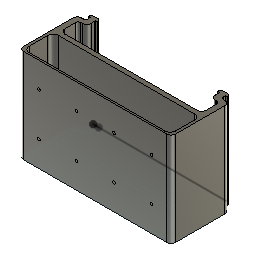
Robot Arm Holder (Autodesk Fusion 360 design; units mm, degrees)
Autodesk Fusion 360 part; units mm, degrees
sketch "Sketch1" plane through (0, 0, 0) normal (0, 0, 1) x (1, 0, 0)
  line L0 (69.451, 50) -> (67.151, 50)
  line L1 (-69.451, 50) -> (-67.151, 50)
  line L2 (-67.151, 50) -> (-67.151, 51)
  line L3 (-67.151, 51) -> (-69.4845, 53.3335)
  line L4 (-67.151, 51) -> (-63.851, 51) construction
  line L5 (-69.4845, 53.3335) -> (-75.6165, 53.3335)
  line L6 (-75.6165, 53.3335) -> (-77.9499, 51)
  line L7 (-75.6165, 53.3335) -> (-72.3165, 53.3335) construction
  line L8 (-77.9499, 51) -> (-77.9499, 50)
  line L9 (-77.9499, 50) -> (-75.6499, 50)
  line L10 (-75.6499, 50) -> (-75.6499, 47.5)
  line L11 (-85, -15) -> (-85, 40)
  arc A0 (-78.1499, 45) -> (-75.6499, 47.5) centre (-78.1499, 47.5) ccw
  arc A1 (-80, 45) -> (-85, 40) centre (-80, 40) ccw
  line L12 (-80, 45) -> (-78.1499, 45)
  line L13 (-80, -20) -> (80, -20)
  line L14 (85, -15) -> (85, 40)
  arc A2 (-85, -15) -> (-80, -20) centre (-80, -15) ccw
  arc A3 (80, -20) -> (85, -15) centre (80, -15) ccw
  arc A4 (85, 40) -> (80, 45) centre (80, 40) ccw
  arc A5 (-79, -12) -> (-76, -15) centre (-76, -12) ccw
  arc A6 (76, -15) -> (79, -12) centre (76, -12) ccw
  line L15 (76, -15) -> (-76, -15)
  arc A7 (-76, 40) -> (-79, 37) centre (-76, 37) ccw
  line L16 (-79, 37) -> (-79, -12)
  line L17 (79, -12) -> (79, 37)
  arc A8 (79, 37) -> (76, 40) centre (76, 37) ccw
  line L18 (80, 45) -> (78.15, 45)
  line L19 (75.65, 47.5) -> (75.65, 50)
  line L20 (75.65, 50) -> (77.95, 50)
  line L21 (77.95, 50) -> (77.95, 51)
  line L22 (77.95, 51) -> (75.6165, 53.3335)
  arc A9 (75.65, 47.5) -> (78.15, 45) centre (78.15, 47.5) ccw
  line L23 (75.6165, 53.3335) -> (69.4845, 53.3335)
  line L24 (69.4845, 53.3335) -> (67.1511, 51)
  line L25 (69.4845, 53.3335) -> (72.7845, 53.3335) construction
  line L26 (67.1511, 51) -> (67.151, 50)
  line L27 (69.451, 50) -> (69.451, 47.5)
  arc A10 (66.951, 45) -> (69.451, 47.5) centre (66.951, 47.5) ccw
  line L28 (-69.451, 50) -> (-69.451, 47.5)
  arc A11 (-69.451, 47.5) -> (-66.951, 45) centre (-66.951, 47.5) ccw
  line L29 (-66.951, 45) -> (66.951, 45)
  line L30 (-76, 40) -> (76, 40)
  dimension "d7" = 2.3
  dimension "d8" = 2.3
  dimension "d10" = 1
  dimension "d11" = 135
  dimension "d12" = 3.3
  dimension "d13" = 6.132
  dimension "d14" = 135
  dimension "d15" = 3.3
  dimension "d16" = 1
  dimension "d17" = 2.3
  dimension "d19" = 1.85
  dimension "d22" = 2.3
  dimension "d23" = 135
  dimension "d24" = 3.3
  dimension "d25" = 6.132
  dimension "d26" = 135
  dimension "d27" = 3.3
  constraint perpendicular L1 L2
  constraint horizontal L4
  constraint horizontal L5
  constraint horizontal L7
  constraint perpendicular L5 L8
  constraint perpendicular L8 L9
  constraint perpendicular L9 L10
  constraint tangent A0 L12
  constraint tangent L14 A4
  constraint tangent A5 L16
  constraint tangent L17 A8
  constraint horizontal L18
  constraint perpendicular L19 L20
  constraint perpendicular L20 L21
  constraint horizontal L23
  constraint horizontal L25
  constraint tangent L27 A10
  constraint perpendicular L1 L28
  constraint tangent A10 L29
  constraint tangent A8 L30
  measures "d7" distance of L0.start L0.end
  measures "d8" distance of L1.start L1.end
  measures "d10" distance of L1.end L2.end
  measures "d11" angle of L3 L4
  measures "d12" distance of L2.end L3.end
  measures "d13" distance of L3.end L5.end
  measures "d14" angle of L6 L7
  measures "d15" distance of L5.end L6.end
  measures "d16" distance of L6.end L8.end
  measures "d17" distance of L8.end L9.end
  measures "d19" distance of A4.end L18.end
  measures "d22" distance of L19.end L20.end
  measures "d23" angle of L21 L22
  measures "d24" distance of L21.end L22.end
  measures "d25" distance of L22.end L23.end
  measures "d26" angle of L24 L25
  measures "d27" distance of L23.end L24.end
extrude "Extrude1" add sketch "Sketch1" along normal blind 53
sketch "Sketch2" plane through (0, -15, 0) normal (0, 1, 0) x (-1, 0, 0)
  line L0 (-76, 0) -> (76, 0)
  line L1 (76, 0) -> (76, 53)
  line L2 (76, 53) -> (-76, 53)
  line L3 (-76, 53) -> (-76, 0)
  line L4 (76, 0) -> (70, 0)
  line L5 (70, 0) -> (70, 3)
  line L6 (70, 3) -> (76, 3)
  line L7 (76, 0) -> (76, 3)
  line L8 (-76, 0) -> (-70, 0)
  line L9 (-70, 0) -> (-70, 3)
  line L10 (-70, 3) -> (-76, 3)
  line L11 (-76, 0) -> (-76, 3)
  line L12 (-70, 0) -> (-76, 0)
  line L13 (-76, 0) -> (-76, 3)
  constraint coincident L0.end L1.start
  constraint coincident L0 L4.end
  constraint perpendicular L1 L4
  constraint perpendicular L4 L5
  constraint coincident L1 L6.end
  constraint perpendicular L1 L6
  constraint coincident L0.start L3.end
  constraint coincident L0 L8.end
  constraint perpendicular L3 L8
  constraint perpendicular L8 L9
  constraint coincident L3 L10.end
  constraint perpendicular L3 L10
extrude "Extrude2" add sketch "Sketch2" along normal blind 5 contours L0 L3 L8 L9 L10 L11 L12 L13
extrude "Extrude3" add sketch "Sketch2" along normal blind 5 contours L0 L1 L4 L5 L6 L7
sketch "Sketch3" plane through (0, 40, 0) normal (0, -1, 0) x (1, 0, 0)
  line L0 (-76, 0) -> (76, 0)
  line L1 (76, 0) -> (76, 53)
  line L2 (76, 53) -> (-76, 53)
  line L3 (-76, 53) -> (-76, 0)
  line L4 (76, 0) -> (70, 0)
  line L5 (70, 0) -> (70, 3)
  line L6 (70, 3) -> (76, 3)
  line L7 (76, 3) -> (76, 0)
  line L8 (-76, 0) -> (-70, 0)
  line L9 (-70, 0) -> (-70, 3)
  line L10 (-70, 3) -> (-76, 3)
  line L11 (-76, 3) -> (-76, 0)
  constraint coincident L0.end L1.start
  constraint coincident L0 L4.end
  constraint perpendicular L1 L4
  constraint perpendicular L4 L5
  constraint coincident L1 L6.end
  constraint perpendicular L1 L6
  constraint coincident L0.start L3.end
  constraint coincident L0 L8.end
  constraint perpendicular L3 L8
  constraint perpendicular L8 L9
  constraint coincident L3 L10.end
  constraint perpendicular L3 L10
extrude "Extrude4" add sketch "Sketch3" along normal blind 5 contours L0 L3 L8 L9 L10 L11
extrude "Extrude5" add sketch "Sketch3" along normal blind 5 contours L0 L1 L4 L5 L6 L7
sketch "Sketch4" plane through (0, 0, 53) normal (0, 0, 1) x (-1, 0, 0)
  line L0 (79, 12) -> (79, -37)
  arc A0 (76, -40) -> (79, -37) centre (76, -37) ccw
  line L1 (76, -40) -> (-76, -40)
  arc A1 (-79, -37) -> (-76, -40) centre (-76, -37) ccw
  line L2 (-79, -37) -> (-79, 12)
  arc A2 (-76, 15) -> (-79, 12) centre (-76, 12) ccw
  line L3 (-76, 15) -> (76, 15)
  arc A3 (79, 12) -> (76, 15) centre (76, 12) ccw
  line L4 (69.451, -50) -> (67.151, -50)
  line L5 (67.151, -50) -> (67.151, -51)
  line L6 (67.151, -51) -> (69.4845, -53.3335)
  line L7 (69.4845, -53.3335) -> (75.6165, -53.3335)
  line L8 (75.6165, -53.3335) -> (77.9499, -51)
  line L9 (77.9499, -51) -> (77.9499, -50)
  line L10 (77.9499, -50) -> (75.6499, -50)
  line L11 (75.6499, -50) -> (75.6499, -47.5)
  arc A4 (78.1499, -45) -> (75.6499, -47.5) centre (78.1499, -47.5) ccw
  line L12 (78.1499, -45) -> (80, -45)
  arc A5 (80, -45) -> (85, -40) centre (80, -40) ccw
  line L13 (85, -40) -> (85, 15)
  arc A6 (85, 15) -> (80, 20) centre (80, 15) ccw
  line L14 (80, 20) -> (-80, 20)
  arc A7 (-80, 20) -> (-85, 15) centre (-80, 15) ccw
  line L15 (-85, 15) -> (-85, -40)
  arc A8 (-85, -40) -> (-80, -45) centre (-80, -40) ccw
  line L16 (-80, -45) -> (-78.15, -45)
  arc A9 (-75.65, -47.5) -> (-78.15, -45) centre (-78.15, -47.5) ccw
  line L17 (-75.65, -47.5) -> (-75.65, -50)
  line L18 (-75.65, -50) -> (-77.95, -50)
  line L19 (-77.95, -50) -> (-77.95, -51)
  line L20 (-77.95, -51) -> (-75.6165, -53.3335)
  line L21 (-75.6165, -53.3335) -> (-69.4845, -53.3335)
  line L22 (-69.4845, -53.3335) -> (-67.1511, -51)
  line L23 (-67.1511, -51) -> (-67.151, -50)
  line L24 (-67.151, -50) -> (-69.451, -50)
  line L25 (-69.451, -50) -> (-69.451, -47.5)
  arc A10 (-66.951, -45) -> (-69.451, -47.5) centre (-66.951, -47.5) ccw
  line L26 (-66.951, -45) -> (66.951, -45)
  arc A11 (69.451, -47.5) -> (66.951, -45) centre (66.951, -47.5) ccw
  line L27 (69.451, -47.5) -> (69.451, -50)
  line L28 (-79, 12) -> (-79, 10)
  line L29 (-79, 10) -> (-79, -5)
  line L30 (-79, -5) -> (-85, -5)
  line L31 (-85, -5) -> (-85, 10)
  line L32 (-85, 10) -> (-79, 10)
  line L33 (-79, -37) -> (-79, -35)
  line L34 (-79, -35) -> (-79, -20)
  line L35 (-79, -20) -> (-85, -20)
  line L36 (-85, -20) -> (-85, -35)
  line L37 (-85, -35) -> (-79, -35)
  line L38 (79, 12) -> (79, 10)
  line L39 (79, 10) -> (79, -5)
  line L40 (79, -5) -> (85, -5)
  line L41 (85, -5) -> (85, 10)
  line L42 (85, 10) -> (79, 10)
  line L43 (79, -37) -> (79, -35)
  line L44 (79, -35) -> (79, -20)
  line L45 (79, -20) -> (85, -20)
  line L46 (85, -20) -> (85, -35)
  line L47 (85, -35) -> (79, -35)
  constraint coincident L2.end A2.end
  constraint coincident L2 L28.end
  constraint parallel L2 L28
  constraint coincident L2 L29.end
  constraint parallel L2 L29
  constraint coincident L15 L30.end
  constraint perpendicular L15 L30
  constraint coincident L15 L31.end
  constraint perpendicular L30 L31
  constraint perpendicular L2 L32
  constraint coincident A1.start L2.start
  constraint coincident L2 L33.end
  constraint parallel L2 L33
  constraint coincident L2 L34.end
  constraint parallel L2 L34
  constraint coincident L15 L35.end
  constraint perpendicular L15 L35
  constraint coincident L15 L36.end
  constraint perpendicular L35 L36
  constraint perpendicular L2 L37
  constraint coincident L0.start A3.start
  constraint coincident L0 L38.end
  constraint perpendicular L37 L38
  constraint coincident L0 L39.end
  constraint parallel L0 L39
  constraint coincident L13 L40.end
  constraint perpendicular L13 L40
  constraint coincident L13 L41.end
  constraint perpendicular L40 L41
  constraint perpendicular L39 L42
  constraint coincident L0.end A0.end
  constraint coincident L0 L43.end
  constraint perpendicular L42 L43
  constraint coincident L0 L44.end
  constraint parallel L0 L44
  constraint coincident L13 L45.end
  constraint perpendicular L13 L45
  constraint coincident L13 L46.end
  constraint perpendicular L45 L46
  constraint perpendicular L44 L47
extrude "Extrude6" cut sketch "Sketch4" against normal blind 10 contours L2 L15 L34 L35 L36 L37
extrude "Extrude7" cut sketch "Sketch4" against normal blind 10 contours L2 L15 L29 L30 L31 L32
extrude "Extrude8" cut sketch "Sketch4" against normal blind 10 contours L0 L13 L44 L45 L46 L47
extrude "Extrude9" cut sketch "Sketch4" against normal blind 10 contours L0 L13 L39 L40 L41 L42
extrude "Extrude10" add sketch "Sketch4" against normal blind 10 contours L2 L15 L34 L35 L36 L37
extrude "Extrude11" add 1 faces at (83, 0, 43) along direction (0, 0, 1) blind 10
extrude "Extrude12" add 1 faces at (-81, -5, 43) along direction (0, 0, 1) blind 10
extrude "Extrude13" cut 1 faces at (74, -10, 2) along direction (0, -1, 0) blind 5
extrude "Extrude14" cut 1 faces at (-72, -10, 2) along direction (0, -1, 0) blind 5
extrude "Extrude15" cut 1 faces at (72, 35, 2) along direction (0, 1, 0) blind 5
extrude "Extrude16" cut 1 faces at (-74, 35, 2) along direction (0, 1, 0) blind 5
extrude "Extrude17" add 1 faces at (-81, 25, 43) along direction (0, 0, 1) blind 10
sketch "Sketch5" plane through (0, 0, 0) normal (0, 0, 1) x (1, 0, 0)
  line L0 (0, -15) -> (0, 15)
  line L1 (0, 15) -> (79, 15)
  line L2 (79, 15) -> (-79, 15)
  line L3 (69.45, 48) -> (69.45, 38.5)
  line L4 (69.45, 38.5) -> (-69, 38.5)
  line L5 (-69.5, 48.5) -> (-69.5, 38.5)
  line L6 (-69.5, 38.5) -> (-69, 38.5)
  line L7 (-69.5, 48.5) -> (69.45, 48.5)
  line L8 (69.45, 48.5) -> (69.45, 48)
  constraint vertical L0
  constraint perpendicular L0 L1
  constraint parallel L1 L2
  constraint vertical L3
  constraint perpendicular L3 L4
  constraint perpendicular L4 L5
  constraint perpendicular L5 L6
  constraint perpendicular L3 L7
  constraint perpendicular L7 L8
extrude "Extrude18" add sketch "Sketch5" against normal blind 100
extrude "Extrude19" cut 1 faces at (-23.1833, 41.8333, -100) along direction (0, 0, 1) blind 200
sketch "Sketch6" plane through (0, 0, 0) normal (0, 0, -1) x (1, 0, 0)
  line L0 (69.45, -40) -> (69.45, -47.4292)
  arc A0 (69.451, -47.5) -> (69.45, -47.4292) centre (66.951, -47.5) ccw
  line L1 (69.451, -47.5) -> (69.451, -50)
  line L2 (69.451, -50) -> (67.151, -50)
  line L3 (67.151, -50) -> (67.1511, -51)
  line L4 (67.1511, -51) -> (69.4845, -53.3335)
  line L5 (69.4845, -53.3335) -> (75.6165, -53.3335)
  line L6 (75.6165, -53.3335) -> (77.95, -51)
  line L7 (77.95, -51) -> (77.95, -50)
  line L8 (77.95, -50) -> (75.65, -50)
  line L9 (75.65, -50) -> (75.65, -47.5)
  arc A1 (78.15, -45) -> (75.65, -47.5) centre (78.15, -47.5) ccw
  line L10 (78.15, -45) -> (80, -45)
  arc A2 (80, -45) -> (85, -40) centre (80, -40) ccw
  line L11 (85, -40) -> (85, 15)
  arc A3 (85, 15) -> (80, 20) centre (80, 15) ccw
  line L12 (80, 20) -> (-80, 20)
  arc A4 (-80, 20) -> (-85, 15) centre (-80, 15) ccw
  line L13 (-85, 15) -> (-85, -40)
  arc A5 (-85, -40) -> (-80, -45) centre (-80, -40) ccw
  line L14 (-80, -45) -> (-78.1499, -45)
  arc A6 (-75.6499, -47.5) -> (-78.1499, -45) centre (-78.1499, -47.5) ccw
  line L15 (-75.6499, -47.5) -> (-75.6499, -50)
  line L16 (-75.6499, -50) -> (-77.9499, -50)
  line L17 (-77.9499, -50) -> (-77.9499, -51)
  line L18 (-77.9499, -51) -> (-75.6165, -53.3335)
  line L19 (-75.6165, -53.3335) -> (-69.4845, -53.3335)
  line L20 (-69.4845, -53.3335) -> (-67.151, -51)
  line L21 (-67.151, -51) -> (-67.151, -50)
  line L22 (-67.151, -50) -> (-69.451, -50)
  line L23 (-69.451, -50) -> (-69.451, -48.5)
  line L24 (-69.451, -48.5) -> (-69.5, -48.5)
  line L25 (-69.5, -48.5) -> (-69.5, -40)
  line L26 (-69.5, -40) -> (-76, -40)
  arc A7 (-79, -37) -> (-76, -40) centre (-76, -37) ccw
  line L27 (-79, -37) -> (-79, 12)
  arc A8 (-76, 15) -> (-79, 12) centre (-76, 12) ccw
  line L28 (-76, 15) -> (76, 15)
  arc A9 (79, 12) -> (76, 15) centre (76, 12) ccw
  line L29 (79, 12) -> (79, -37)
  arc A10 (76, -40) -> (79, -37) centre (76, -37) ccw
  line L30 (76, -40) -> (69.45, -40)
  line L31 (79, -15) -> (79, -20)
  line L32 (79, -20) -> (-79, -20)
  line L33 (-79, -20) -> (-79, -15)
  line L34 (-79, -15) -> (79, -15)
  constraint coincident L29 L31.start
  constraint coincident L29 L31.end
  constraint coincident L27 L32.end
  constraint perpendicular L27 L32
  constraint coincident L27 L33.end
  constraint perpendicular L32 L33
  constraint perpendicular L31 L34
extrude "Extrude20" add sketch "Sketch6" against normal blind 49 contours L27 L29 L31 L32 L33 L34
extrude "Extrude21" add 1 faces at (26.3333, 18.3333, 49) along direction (0, 0, 1) blind 4
extrude "Extrude22" add 1 faces at (-83, 13.3333, 0) along direction (0, 0, -1) blind 47.6
extrude "Extrude23" cut 1 faces at (-83, 13.3333, -47.6) along direction (0, 0, 1) blind 0.6
extrude "Extrude24" add 1 faces at (-83, 13.3333, -47) along direction (0, 0, -1) blind 5
sketch "Sketch7" plane through (0, 0, -52) normal (0, 0, -1) x (1, 0, 0)
  line L0 (79, -20) -> (79, -37)
  arc A0 (76, -40) -> (79, -37) centre (76, -37) ccw
  line L1 (76, -40) -> (69.45, -40)
  line L2 (69.45, -40) -> (69.45, -47.4292)
  arc A1 (69.451, -47.5) -> (69.45, -47.4292) centre (66.951, -47.5) ccw
  line L3 (69.451, -47.5) -> (69.451, -50)
  line L4 (69.451, -50) -> (67.151, -50)
  line L5 (67.151, -50) -> (67.1511, -51)
  line L6 (67.1511, -51) -> (69.4845, -53.3335)
  line L7 (69.4845, -53.3335) -> (75.6165, -53.3335)
  line L8 (75.6165, -53.3335) -> (77.95, -51)
  line L9 (77.95, -51) -> (77.95, -50)
  line L10 (77.95, -50) -> (75.65, -50)
  line L11 (75.65, -50) -> (75.65, -47.5)
  arc A2 (78.15, -45) -> (75.65, -47.5) centre (78.15, -47.5) ccw
  line L12 (78.15, -45) -> (80, -45)
  arc A3 (80, -45) -> (85, -40) centre (80, -40) ccw
  line L13 (85, -40) -> (85, 15)
  arc A4 (85, 15) -> (80, 20) centre (80, 15) ccw
  line L14 (80, 20) -> (-80, 20)
  arc A5 (-80, 20) -> (-85, 15) centre (-80, 15) ccw
  line L15 (-85, 15) -> (-85, -40)
  arc A6 (-85, -40) -> (-80, -45) centre (-80, -40) ccw
  line L16 (-80, -45) -> (-78.1499, -45)
  arc A7 (-75.6499, -47.5) -> (-78.1499, -45) centre (-78.1499, -47.5) ccw
  line L17 (-75.6499, -47.5) -> (-75.6499, -50)
  line L18 (-75.6499, -50) -> (-77.9499, -50)
  line L19 (-77.9499, -50) -> (-77.9499, -51)
  line L20 (-77.9499, -51) -> (-75.6165, -53.3335)
  line L21 (-75.6165, -53.3335) -> (-69.4845, -53.3335)
  line L22 (-69.4845, -53.3335) -> (-67.151, -51)
  line L23 (-67.151, -51) -> (-67.151, -50)
  line L24 (-67.151, -50) -> (-69.451, -50)
  line L25 (-69.451, -50) -> (-69.451, -48.5)
  line L26 (-69.451, -48.5) -> (-69.5, -48.5)
  line L27 (-69.5, -48.5) -> (-69.5, -40)
  line L28 (-69.5, -40) -> (-76, -40)
  arc A8 (-79, -37) -> (-76, -40) centre (-76, -37) ccw
  line L29 (-79, -37) -> (-79, -20)
  line L30 (-79, -20) -> (79, -20)
  line L31 (79, -15) -> (-79, -15)
  line L32 (-79, -15) -> (-79, 12)
  arc A9 (-76, 15) -> (-79, 12) centre (-76, 12) ccw
  line L33 (-76, 15) -> (76, 15)
  arc A10 (79, 12) -> (76, 15) centre (76, 12) ccw
  line L34 (79, 12) -> (79, -15)
  line L35 (-69.5, -40) -> (-69.5, -45)
  line L36 (-69.5, -40) -> (-74.5, -40)
  arc A11 (-69.5, -45) -> (-74.5, -40) centre (-74.5, -45) ccw
  dimension "d78" = 5
  constraint coincident L27.end L28.start
  constraint coincident L27 L35.end
  constraint perpendicular L28 L35
  constraint perpendicular L27 L36
  constraint tangent L27 A11
  measures "d78" distance of L27.end L36.end
extrude "Extrude25" cut sketch "Sketch7" against normal blind 110 contours L27 L28 L35 L36 A11
fillet "Fillet1" radius 5 1 edges at (69.45, 40, 0.5)
sketch "Sketch8" plane through (0, 0, -52) normal (0, 0, -1) x (1, 0, 0)
  line L0 (79, -15) -> (-79, -15)
  line L1 (-79, -15) -> (-79, 12)
  arc A0 (-76, 15) -> (-79, 12) centre (-76, 12) ccw
  line L2 (-76, 15) -> (76, 15)
  arc A1 (79, 12) -> (76, 15) centre (76, 12) ccw
  line L3 (79, 12) -> (79, -15)
  arc A2 (74.45, -40) -> (69.45, -45) centre (74.45, -45) ccw
  line L4 (69.45, -45) -> (69.45, -47.4292)
  arc A3 (69.451, -47.5) -> (69.45, -47.4292) centre (66.951, -47.5) ccw
  line L5 (69.451, -47.5) -> (69.451, -50)
  line L6 (69.451, -50) -> (67.151, -50)
  line L7 (67.151, -50) -> (67.1511, -51)
  line L8 (67.1511, -51) -> (69.4845, -53.3335)
  line L9 (69.4845, -53.3335) -> (75.6165, -53.3335)
  line L10 (75.6165, -53.3335) -> (77.95, -51)
  line L11 (77.95, -51) -> (77.95, -50)
  line L12 (77.95, -50) -> (75.65, -50)
  line L13 (75.65, -50) -> (75.65, -47.5)
  arc A4 (78.15, -45) -> (75.65, -47.5) centre (78.15, -47.5) ccw
  line L14 (78.15, -45) -> (80, -45)
  arc A5 (80, -45) -> (85, -40) centre (80, -40) ccw
  line L15 (85, -40) -> (85, 15)
  arc A6 (85, 15) -> (80, 20) centre (80, 15) ccw
  line L16 (80, 20) -> (-80, 20)
  arc A7 (-80, 20) -> (-85, 15) centre (-80, 15) ccw
  line L17 (-85, 15) -> (-85, -40)
  arc A8 (-85, -40) -> (-80, -45) centre (-80, -40) ccw
  line L18 (-80, -45) -> (-78.1499, -45)
  arc A9 (-75.6499, -47.5) -> (-78.1499, -45) centre (-78.1499, -47.5) ccw
  line L19 (-75.6499, -47.5) -> (-75.6499, -50)
  line L20 (-75.6499, -50) -> (-77.9499, -50)
  line L21 (-77.9499, -50) -> (-77.9499, -51)
  line L22 (-77.9499, -51) -> (-75.6165, -53.3335)
  line L23 (-75.6165, -53.3335) -> (-69.4845, -53.3335)
  line L24 (-69.4845, -53.3335) -> (-67.151, -51)
  line L25 (-67.151, -51) -> (-67.151, -50)
  line L26 (-67.151, -50) -> (-69.451, -50)
  line L27 (-69.451, -50) -> (-69.451, -48.5)
  line L28 (-69.451, -48.5) -> (-69.5, -48.5)
  line L29 (-69.5, -48.5) -> (-69.5, -45)
  arc A10 (-69.5, -45) -> (-74.5, -40) centre (-74.5, -45) ccw
  line L30 (-74.5, -40) -> (-76, -40)
  arc A11 (-79, -37) -> (-76, -40) centre (-76, -37) ccw
  line L31 (-79, -37) -> (-79, -20)
  line L32 (-79, -20) -> (79, -20)
  line L33 (79, -20) -> (79, -37)
  arc A12 (76, -40) -> (79, -37) centre (76, -37) ccw
  line L34 (76, -40) -> (74.45, -40)
  line L35 (0, -20) -> (0, -50)
  constraint midpoint L32 L35.start
  constraint perpendicular L32 L35
sketch "Sketch9" plane through (0, 20, 0) normal (0, 1, 0) x (-1, 0, 0)
  line L0 (79, -52) -> (79, 53)
  line L1 (79, 53) -> (-79, 53)
  line L2 (-79, 53) -> (-79, -52)
  line L3 (-79, -52) -> (79, -52)
  line L4 (0, -52) -> (0, 53)
  line L5 (0, 53) -> (0, 0.5)
  circle A0 centre (0, 0.5) radius 41.5
  line L6 (0, 0) -> (11, 0)
  line L7 (11, 0) -> (11, -20)
  line L8 (0, -41) -> (0, -32.3)
  line L9 (0, -20) -> (0, -32.3)
  line L10 (0, -32.3) -> (11, -32.3)
  line L11 (11, -32.3) -> (11, 7.7)
  line L12 (11, 7.7) -> (-11, 7.7)
  line L13 (-11, 7.7) -> (-11, -32.3)
  line L14 (-11, -32.3) -> (11, -32.3)
  circle A1 centre (-11, 7.7) radius 1.25
  circle A2 centre (11, 7.7) radius 1.25
  circle A3 centre (11, -32.3) radius 1.25
  circle A4 centre (-11, -32.3) radius 1.25
  dimension "d83" = 52.5
  dimension "d84" = 83
  dimension "d107" = 8.7
  dimension "d108" = 40
  dimension "d109" = 40
  dimension "d110" = 2.5
  dimension "d111" = 2.5
  dimension "d112" = 2.5
  dimension "d113" = 2.5
  constraint midpoint L3 L4.start
  constraint midpoint L1 L4.end
  constraint perpendicular L1 L5
  constraint coincident L5.end A0.centre
  constraint coincident L6.start origin
  constraint perpendicular L5 L6
  constraint perpendicular L6 L7
  constraint coincident A0 L8.start
  constraint coincident L4 L8.start
  constraint parallel L4 L8
  constraint perpendicular L4 L10
  constraint perpendicular L6 L11
  constraint perpendicular L11 L12
  constraint perpendicular L12 L13
  constraint perpendicular L11 L14
  constraint coincident L12.end L13.start
  constraint coincident L11.end L12.start
  constraint coincident L10.end L11.start
  constraint coincident L13.end L14.start
  measures "d83" distance of L4.end L5.end
  measures "d84" diameter of A0
  measures "d107" distance of L8.start L8.end
  measures "d108" distance of L10.end L11.end
  measures "d109" distance of L12.end L13.end
  measures "d110" diameter of A1
  measures "d111" diameter of A2
  measures "d112" diameter of A3
  measures "d113" diameter of A4
extrude "Extrude31" cut sketch "Sketch9" against normal blind 5 contours L10 L11 L14 A3 | L10 L11 L14 A3 | L13 L14 A4 | L13 L14 A4 | L11 L12 A2 | L11 L12 A2 | L12 L13 A1 | L12 L13 A1
extrude "Extrude26" cut 1 faces at (25.3333, -15, -17) along direction (0, -1, 0) blind 3
extrude "Extrude27" cut 1 faces at (79, 6, -17) along direction (1, 0, 0) blind 3
extrude "Extrude28" cut 1 faces at (-79, -3, 18) along direction (-1, 0, 0) blind 3
extrude "Extrude29" cut 1 faces at (-80, -12, 18) along direction (0, -1, 0) blind 6
extrude "Extrude30" cut 1 faces at (-79, -14, 18) along direction (1, 0, 0) blind 161
fillet "Fillet2" radius 6 1 edges at (-82, -18, 0.5)
fillet "Fillet3" radius 6 1 edges at (82, -18, 0.5)
fillet "Fillet4" radius 6 1 edges at (-82, 15, 0.5)
fillet "Fillet5" radius 6 1 edges at (82, 15, 0.5)
fillet "Fillet6" radius 5 1 edges at (-79, 20, 0.5)
fillet "Fillet7" radius 5 1 edges at (79, 20, 0.5)
sketch "Sketch10" plane through (0, -20, 0) normal (0, -1, 0) x (1, 0, 0)
  line L0 (80, -52) -> (80, 53)
  line L1 (80, 53) -> (-80, 53)
  line L2 (-80, 53) -> (-80, -52)
  line L3 (-80, -52) -> (80, -52)
  line L4 (0, 53) -> (0, -52)
  line L5 (0, -52) -> (0, 0.5)
  line L6 (0, 0.5) -> (21, 0.5)
  line L7 (21, 0.5) -> (-21, 0.5)
  line L8 (-21, 0.5) -> (-21, 24.5)
  line L9 (-21, 24.5) -> (21, 24.5)
  line L10 (21, 24.5) -> (21, -23.5)
  line L11 (21, -23.5) -> (-21, -23.5)
  line L12 (-21, -23.5) -> (-21, 24.5)
  circle A0 centre (-21, 24.5) radius 1.5
  circle A1 centre (21, 24.5) radius 1.5
  circle A2 centre (21, -23.5) radius 1.5
  circle A3 centre (-21, -23.5) radius 1.5
  dimension "d116" = 52.5
  dimension "d117" = 24
  dimension "d118" = 48
  dimension "d119" = 3
  dimension "d120" = 3
  dimension "d121" = 3
  dimension "d122" = 3
  constraint midpoint L1 L4.start
  constraint midpoint L3 L4.end
  constraint perpendicular L3 L5
  constraint perpendicular L4 L6
  constraint perpendicular L4 L7
  constraint perpendicular L6 L8
  constraint perpendicular L4 L9
  constraint perpendicular L9 L10
  constraint perpendicular L10 L11
  constraint perpendicular L9 L12
  constraint coincident L8.end L9.start
  constraint coincident L9.end L10.start
  constraint coincident L10.end L11.start
  constraint coincident L11.end L12.start
  measures "d116" distance of L4.end L5.end
  measures "d117" distance of L7.end L8.end
  measures "d118" distance of L9.end L10.end
  measures "d119" diameter of A0
  measures "d120" diameter of A1
  measures "d121" diameter of A2
  measures "d122" diameter of A3
extrude "Extrude32" cut sketch "Sketch10" against normal blind 5 contours L10 L11 A2 | L10 L11 A2 | L11 L12 A3 | L11 L12 A3 | L8 L9 L12 A0 | L8 L9 L12 A0 | L9 L10 A1 | L9 L10 A1
sketch "Sketch11" plane through (0, -20, 0) normal (0, -1, 0) x (1, 0, 0)
  circle A0 centre (21, -23.5) radius 1.5
  circle A1 centre (21, 24.5) radius 1.5
  circle A2 centre (-21, -23.5) radius 1.5
  circle A3 centre (-21, 24.5) radius 1.5
  line L0 (80, -52) -> (80, 53)
  line L1 (80, 53) -> (-80, 53)
  line L2 (-80, 53) -> (-80, -52)
  line L3 (-80, -52) -> (80, -52)
  line L4 (75, 24.5) -> (33, 24.5)
  line L5 (33, -23.5) -> (75, -23.5)
  line L6 (-33, -23.5) -> (-33, 24.5)
  line L7 (21, 24.5) -> (63, 24.5)
  line L8 (-63, 24.5) -> (-63, -23.5)
  circle A4 centre (-63, 24.5) radius 1.5
  circle A5 centre (-63, -23.5) radius 1.5
  circle A6 centre (63, -23.5) radius 1.5
  circle A7 centre (63, 24.5) radius 1.5
  dimension "d125" = 48
  dimension "d127" = 3
  dimension "d128" = 3
  dimension "d129" = 3
  dimension "d130" = 3
  constraint coincident A1.centre L7.start
  constraint coincident L4 L7.end
  constraint parallel L4 L7
  constraint coincident L8.start A4.centre
  constraint coincident L8.end A5.centre
  constraint coincident L7.end A7.centre
  measures "d125" distance of L4.end L5.start
  measures "d127" diameter of A4
  measures "d128" diameter of A5
  measures "d129" diameter of A6
  measures "d130" diameter of A7
extrude "Extrude33" cut sketch "Sketch11" against normal blind 4 contours L4 L7 A7 | L4 L7 A7 | L5 A6 | L5 A6 | A4 | A5
sketch "Sketch12" plane through (0, 0, -52) normal (0, 0, -1) x (1, 0, 0)
  arc A0 (74.45, -40) -> (69.45, -45) centre (74.45, -45) ccw
  line L0 (69.45, -45) -> (69.45, -47.4292)
  arc A1 (69.451, -47.5) -> (69.45, -47.4292) centre (66.951, -47.5) ccw
  line L1 (69.451, -47.5) -> (69.451, -50)
  line L2 (69.451, -50) -> (67.151, -50)
  line L3 (67.151, -50) -> (67.1511, -51)
  line L4 (67.1511, -51) -> (69.4845, -53.3335)
  line L5 (69.4845, -53.3335) -> (75.6165, -53.3335)
  line L6 (75.6165, -53.3335) -> (77.95, -51)
  line L7 (77.95, -51) -> (77.95, -50)
  line L8 (77.95, -50) -> (75.65, -50)
  line L9 (75.65, -50) -> (75.65, -47.5)
  arc A2 (78.15, -45) -> (75.65, -47.5) centre (78.15, -47.5) ccw
  line L10 (78.15, -45) -> (80, -45)
  arc A3 (80, -45) -> (85, -40) centre (80, -40) ccw
  line L11 (85, -40) -> (85, 15)
  arc A4 (85, 15) -> (80, 20) centre (80, 15) ccw
  line L12 (80, 20) -> (-80, 20)
  arc A5 (-80, 20) -> (-85, 15) centre (-80, 15) ccw
  line L13 (-85, 15) -> (-85, -40)
  arc A6 (-85, -40) -> (-80, -45) centre (-80, -40) ccw
  line L14 (-80, -45) -> (-78.1499, -45)
  arc A7 (-75.6499, -47.5) -> (-78.1499, -45) centre (-78.1499, -47.5) ccw
  line L15 (-75.6499, -47.5) -> (-75.6499, -50)
  line L16 (-75.6499, -50) -> (-77.9499, -50)
  line L17 (-77.9499, -50) -> (-77.9499, -51)
  line L18 (-77.9499, -51) -> (-75.6165, -53.3335)
  line L19 (-75.6165, -53.3335) -> (-69.4845, -53.3335)
  line L20 (-69.4845, -53.3335) -> (-67.151, -51)
  line L21 (-67.151, -51) -> (-67.151, -50)
  line L22 (-67.151, -50) -> (-69.451, -50)
  line L23 (-69.451, -50) -> (-69.451, -48.5)
  line L24 (-69.451, -48.5) -> (-69.5, -48.5)
  line L25 (-69.5, -48.5) -> (-69.5, -45)
  arc A8 (-69.5, -45) -> (-74.5, -40) centre (-74.5, -45) ccw
  line L26 (-74.5, -40) -> (-76, -40)
  arc A9 (-79, -37) -> (-76, -40) centre (-76, -37) ccw
  line L27 (-79, -37) -> (-79, -25)
  arc A10 (-74, -20) -> (-79, -25) centre (-74, -25) ccw
  line L28 (-74, -20) -> (74, -20)
  arc A11 (79, -25) -> (74, -20) centre (74, -25) ccw
  line L29 (79, -25) -> (79, -37)
  arc A12 (76, -40) -> (79, -37) centre (76, -37) ccw
  line L30 (76, -40) -> (74.45, -40)
  line L31 (-76, 18) -> (76, 18)
  arc A13 (82, 12) -> (76, 18) centre (76, 12) ccw
  line L32 (82, 12) -> (82, -9)
  arc A14 (76, -15) -> (82, -9) centre (76, -9) ccw
  line L33 (76, -15) -> (-76, -15)
  arc A15 (-82, -9) -> (-76, -15) centre (-76, -9) ccw
  line L34 (-82, -9) -> (-82, 12)
  arc A16 (-76, 18) -> (-82, 12) centre (-76, 12) ccw
  line L35 (-69.4845, -53.3335) -> (-75.6165, -53.3335)
  line L36 (-75.6165, -53.3335) -> (-72.5505, -53.3335)
  line L37 (-72.5505, -53.3335) -> (72.5505, -53.3335)
  constraint coincident L19.end L20.start
  constraint coincident L18.end L19.start
  constraint midpoint L19 L36.end
  constraint midpoint L5 L37.end
